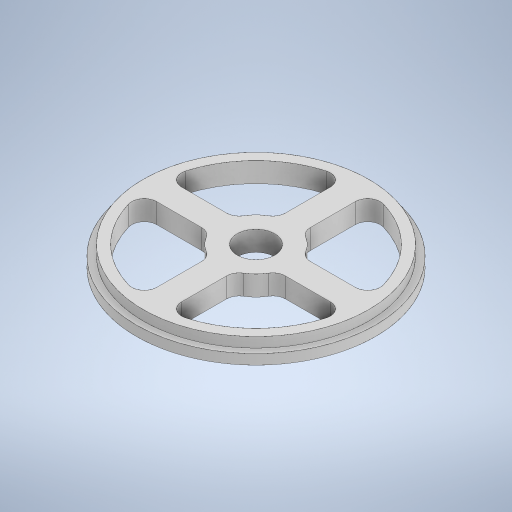
# Autodesk Inventor part: Test_Socle
Saved by Autodesk Inventor 2024 (Build 280153000, 153)
## iProperties
Created: 2025-01-20
Part Number: Test_Socle
Material: Générique
Document SubType Name: Modeling
Designer: malam
Density: 1 g/cm^3
Appearance: Par défaut
Author: malam
Autodesk Inventor part; units mm, degrees
ref_plane "YZ Plane" through (0, 0, 0) normal (1, 0, 0) x (0, 1, 0)
ref_plane "XZ Plane" through (0, 0, 0) normal (0, 1, 0) x (-1, 0, 0)
ref_plane "XY Plane" through (0, 0, 0) normal (0, 0, 1) x (1, 0, 0)
sketch "Esquisse1" plane through (0, 0, 0) normal (0, 1, 0) x (-1, 0, 0)
  circle A0 centre (0, 0) radius 7.5
  circle A1 centre (0, 0) radius 45.155
  circle A2 centre (0, 0) radius 47.86
  dimension "d0" = 15
  dimension "d1" = 90.31
  dimension "d2" = 95.72
  constraints: 3 centre point, 3 coincident
  measures "d0" diameter of A0
  measures "d1" diameter of A1
  measures "d2" diameter of A2
extrude "Extrusion1" add sketch "Esquisse1" along normal blind 4 contours A2
extrude "Extrusion2" add sketch "Esquisse1" along normal blind 8 contours A1
sketch "Esquisse2" plane through (0, 8, 0) normal (0, 1, 0) x (1, 0, 0)
  circle A0 centre (0, 0) radius 45.155 projected
  circle A1 centre (0, 0) radius 7.5 projected
  circle A2 centre (0, 0) radius 14.5
  circle A3 centre (0, 0) radius 41.155
  line L0 (-13.6107, -5) -> (-40.8501, -5)
  line L1 (-14.5, 0) -> (-41.155, 0) construction
  line L2 (-13.6107, 5) -> (-40.8501, 5)
  line L3 (5, -13.6107) -> (5, -40.8501)
  line L4 (-5, -13.6107) -> (-5, -40.8501)
  line L5 (13.6107, 5) -> (40.8501, 5)
  line L6 (13.6107, -5) -> (40.8501, -5)
  line L7 (-5, 13.6107) -> (-5, 40.8501)
  line L8 (5, 13.6107) -> (5, 40.8501)
  dimension "d7" = 7
  dimension "d8" = 4
  dimension "d9" = 5
  dimension "d10" = 5
  dimension "d13" = 360
  constraints: 18 end point, 6 point on circle, 4 horizontal, 2 centre point, 25 other
  measures "d7" radial gap between concentric circles of A1 A2
  measures "d8" radial gap between concentric circles of A0 A3
  measures "d9" distance between parallel lines of L1 L0
  measures "d10" distance between parallel lines of L1 L2
extrude "Extrusion3" cut sketch "Esquisse2" against normal through all contours A2 L8 A3 L5 | L6 A3 L3 A2 | A2 L2 A3 L7 | L4 A3 L0 A2
fillet "Congé1" radius 5 16 edges at (-40.8501, 4, 5) (-5, 4, 40.8501) (5, 4, 40.8501) (-40.8501, 4, -5) (40.8501, 4, 5) (-5, 4, -40.8501) (5, 4, -40.8501) (40.8501, 4, -5) (5, 4, -13.6107) (13.6107, 4, -5) (13.6107, 4, 5) (5, 4, 13.6107) (-5, 4, 13.6107) (-13.6107, 4, 5) (-13.6107, 4, -5) (-5, 4, -13.6107)
sketch "Esquisse3" plane through (0, 0, 0) normal (0, -1, 0) x (1, 0, 0)
  line L0 (16.7407, -5) -> (34.7446, -5) projected
  arc A0 (39.5495, -11.3829) -> (34.7446, -5) centre (34.7446, -10) ccw projected
  arc A1 (11.3829, -39.5495) -> (39.5495, -11.3829) centre (0, 0) ccw projected
  arc A2 (5, -34.7446) -> (11.3829, -39.5495) centre (10, -34.7446) ccw projected
  line L1 (5, -34.7446) -> (5, -16.7407) projected
  arc A3 (7.4359, -12.4482) -> (5, -16.7407) centre (10, -16.7407) ccw projected
  arc A4 (7.4359, -12.4482) -> (12.4482, -7.4359) centre (0, 0) ccw projected
  arc A5 (16.7407, -5) -> (12.4482, -7.4359) centre (16.7407, -10) ccw projected
  line L2 (-34.7446, -5) -> (-16.7407, -5) projected
  arc A6 (-12.4482, -7.4359) -> (-16.7407, -5) centre (-16.7407, -10) ccw projected
  arc A7 (-12.4482, -7.4359) -> (-7.4359, -12.4482) centre (0, 0) ccw projected
  arc A8 (-5, -16.7407) -> (-7.4359, -12.4482) centre (-10, -16.7407) ccw projected
  line L3 (-5, -16.7407) -> (-5, -34.7446) projected
  arc A9 (-11.3829, -39.5495) -> (-5, -34.7446) centre (-10, -34.7446) ccw projected
  arc A10 (-39.5495, -11.3829) -> (-11.3829, -39.5495) centre (0, 0) ccw projected
  arc A11 (-34.7446, -5) -> (-39.5495, -11.3829) centre (-34.7446, -10) ccw projected
  line L4 (5, 16.7407) -> (5, 34.7446) projected
  arc A12 (11.3829, 39.5495) -> (5, 34.7446) centre (10, 34.7446) ccw projected
  arc A13 (39.5495, 11.3829) -> (11.3829, 39.5495) centre (0, 0) ccw projected
  arc A14 (34.7446, 5) -> (39.5495, 11.3829) centre (34.7446, 10) ccw projected
  line L5 (34.7446, 5) -> (16.7407, 5) projected
  arc A15 (12.4482, 7.4359) -> (16.7407, 5) centre (16.7407, 10) ccw projected
  arc A16 (12.4482, 7.4359) -> (7.4359, 12.4482) centre (0, 0) ccw projected
  arc A17 (5, 16.7407) -> (7.4359, 12.4482) centre (10, 16.7407) ccw projected
  line L6 (-16.7407, 5) -> (-34.7446, 5) projected
  arc A18 (-39.5495, 11.3829) -> (-34.7446, 5) centre (-34.7446, 10) ccw projected
  arc A19 (-11.3829, 39.5495) -> (-39.5495, 11.3829) centre (0, 0) ccw projected
  arc A20 (-5, 34.7446) -> (-11.3829, 39.5495) centre (-10, 34.7446) ccw projected
  line L7 (-5, 34.7446) -> (-5, 16.7407) projected
  arc A21 (-7.4359, 12.4482) -> (-5, 16.7407) centre (-10, 16.7407) ccw projected
  arc A22 (-7.4359, 12.4482) -> (-12.4482, 7.4359) centre (0, 0) ccw projected
  arc A23 (-16.7407, 5) -> (-12.4482, 7.4359) centre (-16.7407, 10) ccw projected
  circle A24 centre (0, 0) radius 7.5 projected
  circle A25 centre (0, 0) radius 47.86 projected
  line L8 (0, 0) -> (47.2033, -47.2033) construction
  line L9 (0, 0) -> (66.7555, 0) construction
  line L10 (31.007, -35.3053) -> (26.8664, -30.963)
  line L11 (26.8664, -30.963) -> (31.2086, -26.8224)
  line L12 (31.2086, -26.8224) -> (35.3493, -31.1646)
  line L13 (35.3493, -31.1646) -> (31.007, -35.3053)
  line L14 (31.007, -35.3053) -> (31.2086, -26.8224) construction
  line L15 (26.8664, -30.963) -> (35.3493, -31.1646) construction
  line L16 (26.8224, 31.2086) -> (31.1646, 35.3493)
  line L17 (30.963, 26.8664) -> (31.1646, 35.3493) construction
  line L18 (35.3053, 31.007) -> (30.963, 26.8664)
  line L19 (35.3053, 31.007) -> (26.8224, 31.2086) construction
  line L20 (31.1646, 35.3493) -> (35.3053, 31.007)
  line L21 (30.963, 26.8664) -> (26.8224, 31.2086)
  line L22 (-31.2086, 26.8224) -> (-35.3493, 31.1646)
  line L23 (-26.8664, 30.963) -> (-35.3493, 31.1646) construction
  line L24 (-31.007, 35.3053) -> (-26.8664, 30.963)
  line L25 (-31.007, 35.3053) -> (-31.2086, 26.8224) construction
  line L26 (-35.3493, 31.1646) -> (-31.007, 35.3053)
  line L27 (-26.8664, 30.963) -> (-31.2086, 26.8224)
  line L28 (-26.8224, -31.2086) -> (-31.1646, -35.3493)
  line L29 (-30.963, -26.8664) -> (-31.1646, -35.3493) construction
  line L30 (-35.3053, -31.007) -> (-30.963, -26.8664)
  line L31 (-35.3053, -31.007) -> (-26.8224, -31.2086) construction
  line L32 (-31.1646, -35.3493) -> (-35.3053, -31.007)
  line L33 (-30.963, -26.8664) -> (-26.8224, -31.2086)
  point P0 (31.1078, -31.0638)
  point P1 (31.0521, -31.0521)
  point P2 (31.0638, 31.1078)
  point P3 (31.0521, 31.0521)
  point P4 (-31.1078, 31.0638)
  point P5 (-31.0521, 31.0521)
  point P6 (-31.0638, -31.1078)
  point P7 (-31.0521, -31.0521)
  point P8 (31.0796, 26.9776)
  point P9 (35.0204, 30.7354)
  point P10 (30.7793, 34.9818)
  point P11 (26.8252, 31.2113)
  point P12 (-26.9776, 31.0796)
  point P13 (-30.7354, 35.0204)
  point P14 (-34.9818, 30.7793)
  point P15 (-31.2113, 26.8252)
  point P16 (-31.0796, -26.9776)
  point P17 (-35.0204, -30.7354)
  point P18 (-30.7793, -34.9818)
  point P19 (-26.8252, -31.2113)
  point P20 (34.9818, -30.7793)
  point P21 (31.2113, -26.8252)
  point P22 (26.9776, -31.0796)
  point P23 (30.7354, -35.0204)
  dimension "d18" = 45
  dimension "d20" = 6
  dimension "d21" = 6
  dimension "d24" = 360
  constraints: 52 end point, 2 midpoint, 2 parallel, 1 equal length, 1 horizontal, 1 perpendicular, 1 point on line, 49 other
  measures "d18" angle of L8 L9
  measures "d20" distance of L11.end L12.end
  measures "d21" distance of L10.end L11.end
extrude "Extrusion4" cut sketch "Esquisse3" against normal blind 4 contours L0 A0 A1 L11 L10 A2 L1 A3 A4 A5 | L12 L13 L10 A1 | A1 L10 L11 | L2 A6 A7 A8 L3 A9 A10 L33 L30 A11 | L30 L33 A10 | A10 L28 L32 L30 | L4 A12 A13 L21 L18 A14 L5 A15 A16 A17 | L16 L20 L18 A13 | A13 L18 L21 | L6 A18 A19 L27 L24 A20 L7 A21 A22 A23 | L22 L26 L24 A19 | A19 L24 L27 | A24 | A25
sketch "Esquisse4" plane through (0, 4, 0) normal (0, -1, 0) x (1, 0, 0)
  circle A0 centre (0, 0) radius 47.86
  arc A1 (-12.4482, -7.4359) -> (-16.7407, -5) centre (-16.7407, -10) ccw projected
  arc A2 (-12.4482, -7.4359) -> (-7.4359, -12.4482) centre (0, 0) ccw projected
  arc A3 (-5, -16.7407) -> (-7.4359, -12.4482) centre (-10, -16.7407) ccw projected
  line L0 (-5, -34.7446) -> (-5, -16.7407) projected
  arc A4 (-11.3829, -39.5495) -> (-5, -34.7446) centre (-10, -34.7446) ccw projected
  arc A5 (-39.5495, -11.3829) -> (-11.3829, -39.5495) centre (0, 0) ccw projected
  arc A6 (-34.7446, -5) -> (-39.5495, -11.3829) centre (-34.7446, -10) ccw projected
  line L1 (-16.7407, -5) -> (-34.7446, -5) projected
  arc A7 (7.4359, -12.4482) -> (5, -16.7407) centre (10, -16.7407) ccw projected
  arc A8 (7.4359, -12.4482) -> (12.4482, -7.4359) centre (0, 0) ccw projected
  arc A9 (16.7407, -5) -> (12.4482, -7.4359) centre (16.7407, -10) ccw projected
  line L2 (34.7446, -5) -> (16.7407, -5) projected
  arc A10 (39.5495, -11.3829) -> (34.7446, -5) centre (34.7446, -10) ccw projected
  arc A11 (11.3829, -39.5495) -> (39.5495, -11.3829) centre (0, 0) ccw projected
  arc A12 (5, -34.7446) -> (11.3829, -39.5495) centre (10, -34.7446) ccw projected
  line L3 (5, -16.7407) -> (5, -34.7446) projected
  arc A13 (34.7446, 5) -> (39.5495, 11.3829) centre (34.7446, 10) ccw projected
  line L4 (16.7407, 5) -> (34.7446, 5) projected
  arc A14 (12.4482, 7.4359) -> (16.7407, 5) centre (16.7407, 10) ccw projected
  arc A15 (12.4482, 7.4359) -> (7.4359, 12.4482) centre (0, 0) ccw projected
  arc A16 (5, 16.7407) -> (7.4359, 12.4482) centre (10, 16.7407) ccw projected
  line L5 (5, 34.7446) -> (5, 16.7407) projected
  arc A17 (11.3829, 39.5495) -> (5, 34.7446) centre (10, 34.7446) ccw projected
  arc A18 (39.5495, 11.3829) -> (11.3829, 39.5495) centre (0, 0) ccw projected
  arc A19 (-5, 34.7446) -> (-11.3829, 39.5495) centre (-10, 34.7446) ccw projected
  line L6 (-5, 16.7407) -> (-5, 34.7446) projected
  arc A20 (-7.4359, 12.4482) -> (-5, 16.7407) centre (-10, 16.7407) ccw projected
  arc A21 (-7.4359, 12.4482) -> (-12.4482, 7.4359) centre (0, 0) ccw projected
  arc A22 (-16.7407, 5) -> (-12.4482, 7.4359) centre (-16.7407, 10) ccw projected
  line L7 (-34.7446, 5) -> (-16.7407, 5) projected
  arc A23 (-39.5495, 11.3829) -> (-34.7446, 5) centre (-34.7446, 10) ccw projected
  arc A24 (-11.3829, 39.5495) -> (-39.5495, 11.3829) centre (0, 0) ccw projected
  circle A25 centre (0, 0) radius 45.155 projected
  circle A26 centre (0, 0) radius 7.5 projected
  dimension "d28" = 95.72
  constraints: 1 centre point, 1 coincident
  measures "d28" diameter of A0
extrude "Extrusion5" add sketch "Esquisse4" along normal blind 4 contours A0 | A25
sketch "Esquisse5" plane through (0, 8, 0) normal (0, 1, 0) x (1, 0, 0)
  line L0 (34.7446, 5) -> (16.7407, 5) projected
  arc A0 (12.4482, 7.4359) -> (16.7407, 5) centre (16.7407, 10) ccw projected
  arc A1 (12.4482, 7.4359) -> (7.4359, 12.4482) centre (0, 0) ccw projected
  arc A2 (5, 16.7407) -> (7.4359, 12.4482) centre (10, 16.7407) ccw projected
  line L1 (5, 16.7407) -> (5, 34.7446) projected
  arc A3 (11.3829, 39.5495) -> (5, 34.7446) centre (10, 34.7446) ccw projected
  arc A4 (39.5495, 11.3829) -> (11.3829, 39.5495) centre (0, 0) ccw projected
  arc A5 (34.7446, 5) -> (39.5495, 11.3829) centre (34.7446, 10) ccw projected
  line L2 (-16.7407, 5) -> (-34.7446, 5) projected
  arc A6 (-39.5495, 11.3829) -> (-34.7446, 5) centre (-34.7446, 10) ccw projected
  arc A7 (-11.3829, 39.5495) -> (-39.5495, 11.3829) centre (0, 0) ccw projected
  arc A8 (-5, 34.7446) -> (-11.3829, 39.5495) centre (-10, 34.7446) ccw projected
  line L3 (-5, 34.7446) -> (-5, 16.7407) projected
  arc A9 (-7.4359, 12.4482) -> (-5, 16.7407) centre (-10, 16.7407) ccw projected
  arc A10 (-7.4359, 12.4482) -> (-12.4482, 7.4359) centre (0, 0) ccw projected
  arc A11 (-16.7407, 5) -> (-12.4482, 7.4359) centre (-16.7407, 10) ccw projected
  line L4 (5, -34.7446) -> (5, -16.7407) projected
  arc A12 (7.4359, -12.4482) -> (5, -16.7407) centre (10, -16.7407) ccw projected
  arc A13 (7.4359, -12.4482) -> (12.4482, -7.4359) centre (0, 0) ccw projected
  arc A14 (16.7407, -5) -> (12.4482, -7.4359) centre (16.7407, -10) ccw projected
  line L5 (16.7407, -5) -> (34.7446, -5) projected
  arc A15 (39.5495, -11.3829) -> (34.7446, -5) centre (34.7446, -10) ccw projected
  arc A16 (11.3829, -39.5495) -> (39.5495, -11.3829) centre (0, 0) ccw projected
  arc A17 (5, -34.7446) -> (11.3829, -39.5495) centre (10, -34.7446) ccw projected
  line L6 (-34.7446, -5) -> (-16.7407, -5) projected
  arc A18 (-12.4482, -7.4359) -> (-16.7407, -5) centre (-16.7407, -10) ccw projected
  arc A19 (-12.4482, -7.4359) -> (-7.4359, -12.4482) centre (0, 0) ccw projected
  arc A20 (-5, -16.7407) -> (-7.4359, -12.4482) centre (-10, -16.7407) ccw projected
  line L7 (-5, -16.7407) -> (-5, -34.7446) projected
  arc A21 (-11.3829, -39.5495) -> (-5, -34.7446) centre (-10, -34.7446) ccw projected
  arc A22 (-39.5495, -11.3829) -> (-11.3829, -39.5495) centre (0, 0) ccw projected
  arc A23 (-34.7446, -5) -> (-39.5495, -11.3829) centre (-34.7446, -10) ccw projected
  circle A24 centre (0, 0) radius 45.155 projected
  circle A25 centre (0, 0) radius 7.5 projected
  circle A26 centre (0, 0) radius 45.305
  dimension "d31" = 0.15
  constraints: 1 centre point
  measures "d31" radial gap between concentric circles of A24 A26
extrude "Extrusion6" add sketch "Esquisse5" against normal up to surface (4 mm away)
extrude "Extrusion7" cut sketch "Esquisse5" against normal up to surface (4 mm away)
